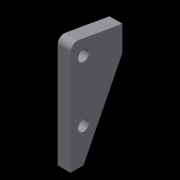
# Autodesk Inventor part: Knuckle
Saved by Autodesk Inventor 2015 (Build 190159000, 159)
## iProperties
RuleStatus: InUse
Created: 2014-10-27
Part Number: Knuckle
Material: Generic
Document SubType Name: Modeling
Designer: Inventor
Mass: 0.622616 g
Surface Area: 6.60895 cm^2
Volume: 0.622616 cm^3
Density: 1 g/cm^3
Appearance: Default
BeforeDocSave0: UpdateBoundingBox
CX: 3.00 mm
CY: 12.00 mm
CZ: 25.71 mm
Author: Inventor
Autodesk Inventor part; units mm, degrees
ref_plane "YZ Plane" through (0, 0, 0) normal (1, 0, 0) x (0, 1, 0)
ref_plane "XZ Plane" through (0, 0, 0) normal (0, 1, 0) x (-1, 0, 0)
ref_plane "XY Plane" through (0, 0, 0) normal (0, 0, 1) x (1, 0, 0)
sketch "Base" plane through (0, 0, 0) normal (1, 0, 0) x (0, 1, 0)
  line L0 (3, -26) -> (0, -26)
  line L1 (3, -26) -> (12, -7.9488)
  line L2 (12, -7.9488) -> (12, -2.1159)
  line L3 (12, -2.1159) -> (0, 0)
  line L4 (0, -26) -> (0, 0)
  dimension "d0" = 12
  dimension "d1" = 80
  dimension "d2" = 26.5
  dimension "d3" = 26
  dimension "d4" = 3
  constraints: 10 end point, 1 coincident, 1 perpendicular, 1 vertical
  measures "d0" distance between parallel lines of L2 L4
  measures "d1" angle of L3 L4
  measures "d2" angle of L1 L4
  measures "d3" distance of L0.end L3.end
  measures "d4" distance of L0.start L0.end
extrude "BaseFeature" add sketch "Base" along normal blind 3
fillet "BaseFilletsFeature" radius 1.5 1 edges at (1.5, 0, 0)
sketch "BaseHoles" plane through (0, 0, 0) normal (-1, 0, 0) x (0, 0, 1)
  line L0 (-26, 3) -> (-0.529, 3) construction
  line L1 (-0.3104, 1.7605) -> (-2.1159, 12) construction
  circle A0 centre (-18.029, 3) radius 1.75
  circle A1 centre (-4.029, 3) radius 1.75
  circle A2 centre (-18.029, 3) radius 7 construction
  circle A3 centre (-4.029, 3) radius 7 construction
  dimension "d9" = 3.5
  dimension "d12" = 3.5
  dimension "d14" = 14
  dimension "d22" = 14
  constraints: 4 centre point, 3 equal radius, 3 point on line, 2 coincident, 2 end point, 1 horizontal
  measures "d9" diameter of A0
  measures "d12" distance of L0.end A1.centre
  measures "d14" diameter of A3
  measures "d22" distance of A0.centre A1.centre
hole "BaseHolesFeature" at (0, 3, -18.029) at (0, 3, -4.029) direction (1, 0, 0) diameter 2.5 end through all
body "Solid1"
